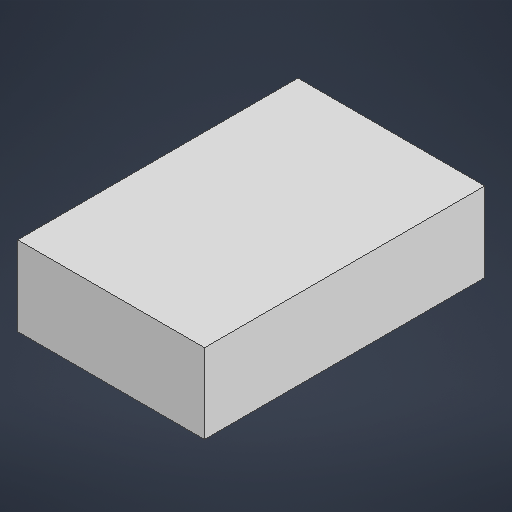
# Autodesk Inventor part: rasberry
Saved by Autodesk Inventor 2025.2 (Build 292293000, 293)
## iProperties
Created: 2024-12-17
Part Number: rasberry
Material: Generic
Document SubType Name: Modeling
Designer: antem
Density: 1 g/cm^3
Appearance: Default
Author: antem
Autodesk Inventor part; units mm, degrees
ref_plane "YZ Plane" through (0, 0, 0) normal (1, 0, 0) x (0, 1, 0)
ref_plane "XZ Plane" through (0, 0, 0) normal (0, 1, 0) x (-1, 0, 0)
ref_plane "XY Plane" through (0, 0, 0) normal (0, 0, 1) x (1, 0, 0)
sketch "Sketch2" plane through (0, 0, 0) normal (0, 0, 1) x (1, 0, 0)
  line L0 (-29.4, 44.095) -> (29.4, 44.095)
  line L1 (29.4, 44.095) -> (29.4, -44.095)
  line L2 (29.4, -44.095) -> (-29.4, -44.095)
  line L3 (-29.4, -44.095) -> (-29.4, 44.095)
  point P0 (0, 0)
  point P1 (29.4, 0)
  point P2 (0, 44.095)
  dimension "d0" = 58.8
  dimension "d1" = 88.19
  constraints: 8 end point, 2 midpoint, 2 parallel, 1 horizontal, 1 horizontal alignment, 1 perpendicular, 1 vertical alignment
  measures "d0" distance of L0.start L0.end
  measures "d1" distance of L2.end L0.start
extrude "Extrusion1" add sketch "Sketch2" along normal blind 25
sketch "Sketch3" plane through (-29.4, 44.095, 0) normal (0, 1, 0) x (1, 0, 0)
  line L0 (23.9, -8) -> (34.9, -8)
  line L1 (34.9, -8) -> (34.9, -7)
  line L2 (34.9, -7) -> (23.9, -7)
  line L3 (23.9, -7) -> (23.9, -8)
  line L4 (58.8, 0) -> (0, 0) projected
  point P0 (29.4, 0)
  point P1 (29.4, 0)
  point P2 (29.4, -7)
  dimension "d4" = 11
  dimension "d5" = 1
  dimension "d6" = 7
  constraints: 8 end point, 2 midpoint, 2 parallel, 1 horizontal, 1 perpendicular, 1 vertical alignment
  measures "d4" distance of L1.end L2.end
  measures "d5" distance of L2.end L0.start
  measures "d6" distance between parallel lines of L4 L2
extrude "Extrusion2" add sketch "Sketch3" along normal blind 3
body "Solid1"
